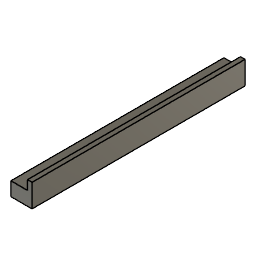
right engine cover part 2 (Autodesk Fusion 360 design; units mm, degrees)
Autodesk Fusion 360 part; units mm, degrees
sketch "Szkic1" plane through (0, 0, 0) normal (0, 0, 1) x (1, 0, 0)
  line L0 (45, 110) -> (-35, 110)
  line L1 (-35, 110) -> (-35, -120)
  line L2 (-35, -120) -> (-29, -120)
  line L3 (-29, -120) -> (-29, -160)
  line L4 (-29, -160) -> (45, -160)
  circle A0 centre (-15, -150) radius 3.5
  circle A1 centre (-15, -130) radius 3.5
  circle A2 centre (20, -130) radius 3.5
  circle A3 centre (20, -150) radius 3.5
  line L5 (-10, -125) -> (10, -125)
  circle A4 centre (-25, -100) radius 1.75
  line L6 (-10, -149) -> (-10, -125)
  circle A5 centre (-25, -50) radius 1.75
  circle A6 centre (-25, 0) radius 1.75
  circle A7 centre (-25, 50) radius 1.75
  circle A8 centre (-25, 100) radius 1.75
  circle A9 centre (25, 100) radius 1.75
  line L7 (-35, 110) -> (-35, 85)
  line L8 (-35, 85) -> (45, 85)
  line L9 (45, 85) -> (45, 110)
  line L10 (45, 110) -> (-35, 110)
  line L11 (-35, 85) -> (-35, -120)
  line L12 (-35, -120) -> (-17, -120)
  line L13 (-17, -120) -> (-17, 85)
  line L14 (-17, 85) -> (-35, 85)
  line L15 (-17, 85) -> (-12, 85)
  line L16 (-12, 85) -> (-12, -120)
  line L17 (-12, -120) -> (-17, -120)
  line L18 (-17, -120) -> (-17, 85)
  dimension "d1" = 18
  constraint perpendicular L7 L8
  constraint parallel L7 L9
  constraint parallel L8 L10
  constraint perpendicular L0 L7
  constraint perpendicular L11 L12
  constraint parallel L11 L13
  constraint parallel L12 L14
  constraint perpendicular L2 L11
  constraint perpendicular L15 L16
  constraint parallel L15 L17
  constraint parallel L16 L18
  constraint perpendicular L13 L15
  measures "d1" distance of L7.end L13.end
extrude "Wyciągnięcie proste1" add sketch "Szkic1" along normal blind 15 contours L1 L2 L8 L11 L12 L13 L14 L18
extrude "Wyciągnięcie proste2" add sketch "Szkic1" along normal blind 25 contours L8 L13 L15 L16 L17 L18
extrude "Wyciągnięcie proste3" add 1 faces at (-21.3333, 85, 5) along direction (0, 1, 0) blind 26
extrude "Wyciągnięcie proste4" cut sketch "Szkic1" along normal blind 38 contours A8
sketch "Szkic2" plane through (0, 0, 0) normal (0, 0, -1) x (1, 0, 0)
  circle A0 centre (-25, -100) radius 1.75
  circle A1 centre (-25, 100) radius 1.75
  circle A2 centre (-25, -50) radius 1.75
  circle A3 centre (-25, 0) radius 1.75
  circle A4 centre (-25, 50) radius 1.75
  line L0 (-12, 120) -> (-35, 120)
  line L1 (-35, 120) -> (-35, -111)
  line L2 (-35, -111) -> (-12, -111)
  line L3 (-12, -111) -> (-12, 120)
  circle A5 centre (-25, -100) radius 3.5
  circle A6 centre (-25, -100) radius 2
  circle A7 centre (-25, -50) radius 2
  circle A8 centre (-25, 0) radius 2
  circle A9 centre (-25, 50) radius 2
  circle A10 centre (-25, 100) radius 2
  dimension "d10" = 7
  dimension "d11" = 4
  dimension "d12" = 4
  dimension "d13" = 4
  dimension "d14" = 4
  dimension "d15" = 4
  constraint concentric A0 A5
  constraint concentric A5 A6
  constraint concentric A2 A7
  constraint concentric A3 A8
  constraint concentric A4 A9
  constraint concentric A1 A10
  measures "d10" diameter of A5
  measures "d11" diameter of A6
  measures "d12" diameter of A7
  measures "d13" diameter of A8
  measures "d14" diameter of A9
  measures "d15" diameter of A10
extrude "Wyciągnięcie proste5" cut sketch "Szkic2" against normal blind 100 contours A6 | A7 | A8 | A9 | A10
extrude "Wyciągnięcie proste6" cut sketch "Szkic2" against normal blind 4 contours A5
